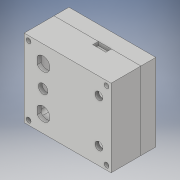
# Autodesk Inventor part: HC_box_v1
Saved by Autodesk Inventor 2018 (Build 220112000, 112)
## iProperties
Created: 2017-06-15
Part Number: HC_box_v1
Material: Generic
Document SubType Name: Modeling
Designer: boss
Density: 1 g/cm^3
Appearance: Default
Author: boss
Autodesk Inventor part; units mm, degrees
ref_plane "YZ Plane" through (0, 0, 0) normal (1, 0, 0) x (0, 1, 0)
ref_plane "XZ Plane" through (0, 0, 0) normal (0, 1, 0) x (-1, 0, 0)
sketch "Sketch1" plane through (0, 0, 0) normal (0, 0, 1) x (1, 0, 0)
  line L0 (-29.591, -26.416) -> (29.591, -26.416)
  line L1 (29.591, -26.416) -> (29.591, 26.416)
  line L2 (29.591, 26.416) -> (-29.591, 26.416)
  line L3 (-29.591, 26.416) -> (-29.591, -26.416)
  line L4 (-29.591, -26.416) -> (29.591, 26.416) construction
  line L5 (29.591, -26.416) -> (-29.591, 26.416) construction
  point P0 (0, 0)
  dimension "d0" = 59.182
  dimension "d1" = 52.832
  constraints: 12 end point, 2 midpoint, 2 parallel, 1 horizontal, 1 perpendicular
  measures "d0" distance of L2.end L1.end
  measures "d1" distance of L1.end L0.end
extrude "Extrusion1" add sketch "Sketch1" along normal blind 2.54
sketch "Sketch2" plane through (0, 0, 2.54) normal (0, 0, 1) x (1, 0, 0)
  line L0 (-27.051, -23.876) -> (27.051, -23.876)
  line L1 (27.051, -23.876) -> (27.051, 23.876)
  line L2 (27.051, 23.876) -> (-27.051, 23.876)
  line L3 (-27.051, 23.876) -> (-27.051, -23.876)
  line L4 (-27.051, -23.876) -> (27.051, 23.876) construction
  line L5 (27.051, -23.876) -> (-27.051, 23.876) construction
  line L6 (29.591, 26.416) -> (-29.591, 26.416) projected
  line L7 (29.591, -26.416) -> (29.591, 26.416) projected
  line L8 (-29.591, -26.416) -> (29.591, -26.416)
  line L9 (29.591, -26.416) -> (29.591, 26.416)
  line L10 (29.591, 26.416) -> (-29.591, 26.416)
  line L11 (-29.591, 26.416) -> (-29.591, -26.416)
  line L12 (-29.591, -26.416) -> (29.591, 26.416) construction
  line L13 (29.591, -26.416) -> (-29.591, 26.416) construction
  line L14 (25.7048, 21.971) -> (-25.7048, 21.971) construction
  line L15 (-25.7048, 21.971) -> (-25.7048, -21.971) construction
  line L16 (-25.7048, -21.971) -> (25.7048, -21.971) construction
  line L17 (25.7048, -21.971) -> (25.7048, 21.971) construction
  line L18 (25.7048, 21.971) -> (-25.7048, -21.971) construction
  line L19 (-25.7048, 21.971) -> (25.7048, -21.971) construction
  point P0 (0, 0)
  dimension "d4" = 2.54
  dimension "d5" = 2.54
  dimension "d39" = 51.4096
  dimension "d40" = 43.942
  constraints: 36 end point, 6 midpoint, 6 parallel, 3 horizontal, 3 perpendicular
  measures "d4" distance between parallel lines of L6 L2
  measures "d5" distance between parallel lines of L7 L1
  measures "d39" distance of L16.end L15.end
  measures "d40" distance of L15.end L14.end
extrude "Extrusion2" add sketch "Sketch2" along normal blind 25.4
sketch "Sketch3" plane through (-29.591, 26.416, 0) normal (0, 1, 0) x (1, 0, 0)
  line L0 (39.116, -10.16) -> (30.226, -10.16)
  line L1 (30.226, -10.16) -> (30.226, -13.97)
  line L2 (30.226, -13.97) -> (39.116, -13.97)
  line L3 (39.116, -13.97) -> (39.116, -10.16)
  line L4 (39.116, -10.16) -> (30.226, -13.97) construction
  line L5 (30.226, -10.16) -> (39.116, -13.97) construction
  line L6 (59.182, 0) -> (0, 0) projected
  line L7 (0, 0) -> (0, -27.94) projected
  line L8 (29.591, 0) -> (29.591, -27.94) construction
  line L9 (56.642, -27.94) -> (2.54, -27.94) construction
  point P0 (34.671, -12.065)
  dimension "d8" = 10.16
  dimension "d10" = 5.08
  dimension "d11" = 8.89
  dimension "d12" = 3.81
  constraints: 14 end point, 3 midpoint, 2 parallel, 1 horizontal, 1 perpendicular
  measures "d8" distance between parallel lines of L6 L0
  measures "d10" distance from line of L8 point (34.671, -12.065)
  measures "d11" distance of L1.end L2.end
  measures "d12" distance of L0.end L1.end
extrude "Extrusion3" cut sketch "Sketch3" against normal up to surface (2.54 mm away)
ref_plane "Work Plane1" through (0, 0, 10.16) normal (0, 0, 1) x (1, 0, 0)
sketch "Sketch4" plane through (0, 0, 27.94) normal (0, 0, 1) x (1, 0, 0)
  line L0 (29.591, 26.416) -> (-29.591, 26.416) projected
  line L1 (29.591, -26.416) -> (-29.591, -26.416)
  line L2 (-29.591, -26.416) -> (-29.591, 26.416)
  line L3 (-29.591, 26.416) -> (29.591, 26.416)
  line L4 (29.591, 26.416) -> (29.591, -26.416)
  line L5 (29.591, -26.416) -> (-29.591, 26.416) construction
  line L6 (-29.591, -26.416) -> (29.591, 26.416) construction
  point P0 (0, 0)
  constraints: 12 end point, 2 midpoint, 2 parallel, 1 horizontal, 1 perpendicular
extrude "Extrusion4" add sketch "Sketch4" along normal blind 2.54
sketch "Sketch5" plane through (0, 0, 30.48) normal (0, 0, 1) x (1, 0, 0)
  circle A0 centre (-16.6948, 14.7623) radius 4.6355
  line L0 (13.97, 21.59) -> (-3.81, 21.59)
  line L1 (-3.81, 21.59) -> (-3.81, -21.59)
  line L2 (-3.81, -21.59) -> (13.97, -21.59)
  line L3 (13.97, -21.59) -> (13.97, 21.59)
  line L4 (13.97, 21.59) -> (-3.81, -21.59) construction
  line L5 (-3.81, 21.59) -> (13.97, -21.59) construction
  line L6 (-41.4274, 0) -> (41.4274, 0) projected
  circle A1 centre (-16.6948, 0) radius 3.2512
  line L7 (-20.6445, 12.3358) -> (-20.6445, 17.1887)
  circle A2 centre (-16.6948, -14.7623) radius 4.6355
  line L8 (-20.6445, -12.3358) -> (-20.6445, -17.1887)
  circle A3 centre (21.3137, 14.7623) radius 2.667
  circle A4 centre (21.3137, -14.7623) radius 2.667
  point P0 (0, 0)
  point P1 (5.08, 0)
  dimension "d18" = 9.271
  dimension "d19" = 17.78
  dimension "d21" = 6.5024
  dimension "d22" = 8.5852
  dimension "d23" = 5.334
  dimension "d41" = 43.18
  dimension "d42" = 5.08
  constraints: 16 end point, 5 centre point, 4 point on circle, 4 symmetric about line, 2 midpoint, 2 parallel, 2 point on line, 1 horizontal, 1 perpendicular, 1 vertical, 2 other
  measures "d18" diameter of A0
  measures "d19" distance of L2.end L1.end
  measures "d21" diameter of A1
  measures "d23" diameter of A3
  measures "d41" distance of L2.end L0.start
  measures "d42" distance of point (0, 0) point (5.08, 0)
extrude "Extrusion5" cut sketch "Sketch5" against normal blind 2.54 contours A0 L7 | A1 L6 | L6 A1 | A2 L8 | A3 | A4 picked at (-15.6636, 16.0265) picked at (-15.4592, -13.8667)
sketch "Sketch6" plane through (0, 0, 2.54) normal (0, 0, 1) x (1, 0, 0)
  circle A0 centre (0, -17.78) radius 1.8415
  line L0 (-41.4274, 0) -> (41.4274, 0) projected
  circle A1 centre (0, 17.78) radius 1.8415
  point P0 (0, 0)
  dimension "d26" = 3.683
  dimension "d27" = 35.56
  constraints: 2 centre point, 1 symmetric about line, 1 other
  measures "d26" diameter of A0
  measures "d27" distance of A1.centre A0.centre
extrude "Extrusion6" cut sketch "Sketch6" against normal blind 2.54
sketch "Sketch7" plane through (0, 0, 30.48) normal (0, 0, 1) x (1, 0, 0)
  line L0 (-29.591, 26.416) -> (-29.591, -26.416) projected
  line L1 (-29.591, -26.416) -> (29.591, -26.416) projected
  line L2 (-41.4274, 0) -> (41.4274, 0) projected
  line L3 (0, 36.9824) -> (0, -36.9824) projected
  point P0 (0, 0)
  point P1 (-26.543, -23.368)
  point P2 (-26.543, 23.368)
  point P3 (26.543, -23.368)
  point P4 (26.543, 23.368)
  dimension "d30" = 3.048
  dimension "d31" = 3.048
  constraints: 3 symmetric about line
  measures "d30" distance from line of L0 point (-26.543, -23.368)
  measures "d31" distance from line of L1 point (-26.543, -23.368)
hole "Hole1" at (-26.543, -23.368, 30.48) at (26.543, -23.368, 30.48) at (26.543, 23.368, 30.48) at (-26.543, 23.368, 30.48) direction (0, 0, -1) diameter 3.2766 end through all clearance for "Flat Head Machine Screw (82)" size "#4" standard "Ansi Unified Screw Threads"
split body "Split2" result two bodies by plane through (0, 0, 10.16) normal (0, 0, 1) first body at (8.3971, 0, 29.98)
body "Solid4"
body "Solid5"
